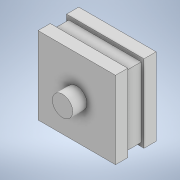
# Autodesk Inventor part: rev motor
Saved by Autodesk Inventor 2022 (Build 260153000, 153)
## iProperties
Created: 2021-07-08
Part Number: rev motor
Material: Generic
Document SubType Name: Modeling
Designer: User
Density: 1 g/cm^3
Appearance: Default
Author: User
Autodesk Inventor part; units mm, degrees
ref_plane "YZ Plane" through (0, 0, 0) normal (1, 0, 0) x (0, 1, 0)
ref_plane "XZ Plane" through (0, 0, 0) normal (0, 1, 0) x (-1, 0, 0)
ref_plane "XY Plane" through (0, 0, 0) normal (0, 0, 1) x (1, 0, 0)
sketch "Sketch1" plane through (0, 0, 0) normal (0, 0, 1) x (1, 0, 0)
  line L0 (-42.8727, 26.6374) -> (-4.7727, 26.6374)
  line L1 (-4.7727, 26.6374) -> (-4.7727, -11.4626)
  line L2 (-4.7727, -11.4626) -> (-42.8727, -11.4626)
  line L3 (-42.8727, -11.4626) -> (-42.8727, 26.6374)
  point P0 (0, 0)
  dimension "d0" = 38.1
  dimension "d1" = 38.1
  constraints: 8 end point, 2 parallel, 1 horizontal, 1 perpendicular
  measures "d0" distance of L1.end L2.end
  measures "d1" distance of L0.end L1.end
extrude "Extrusion1" add sketch "Sketch1" along normal blind 6
sketch "Sketch2" plane through (0, 0, 6) normal (0, 0, 1) x (1, 0, 0)
  line L0 (-41.7124, 24.7081) -> (-6.0889, 24.7081)
  line L1 (-6.0889, 24.7081) -> (-6.0889, -9.5927)
  line L2 (-6.0889, -9.5927) -> (-41.7124, -9.5927)
  line L3 (-41.7124, -9.5927) -> (-41.7124, 24.7081)
  point P0 (0, 0)
  constraints: 8 end point, 2 parallel, 1 horizontal, 1 perpendicular
extrude "Extrusion2" add sketch "Sketch2" along normal blind 8
sketch "Sketch3" plane through (0, 0, 14) normal (0, 0, 1) x (1, 0, 0)
  line L0 (-4.7727, 26.6374) -> (-42.8727, 26.6374) projected
  line L1 (-4.7727, -11.4626) -> (-4.7727, 26.6374) projected
  line L2 (-42.8727, 26.6374) -> (-4.7727, 26.6374)
  line L3 (-4.7727, 26.6374) -> (-4.7727, -11.4626)
  line L4 (-4.7727, -11.4626) -> (-42.8727, -11.4626)
  line L5 (-42.8727, -11.4626) -> (-42.8727, 26.6374)
  point P0 (0, 0)
  constraints: 8 end point, 2 parallel, 1 horizontal, 1 perpendicular
extrude "Extrusion3" add sketch "Sketch3" along normal blind 6
sketch "Sketch4" plane through (0, 0, 20) normal (0, 0, 1) x (1, 0, 0)
  circle A0 centre (-23.8227, 7.5874) radius 5
  line L0 (-4.7727, 26.6374) -> (-42.8727, 26.6374) projected
  line L1 (-4.7727, -11.4626) -> (-4.7727, 26.6374) projected
  point P0 (0, 0)
  dimension "d8" = 10
  dimension "d9" = 19.05
  dimension "d10" = 19.05
  constraints: 1 centre point
  measures "d8" diameter of A0
  measures "d9" distance from line of L0 A0.centre
  measures "d10" distance from line of L1 A0.centre
extrude "Extrusion4" add sketch "Sketch4" along normal blind 7
body "Solid1"
